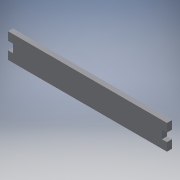
# Autodesk Inventor part: задняя
Saved by Autodesk Inventor 2019 (Build 230136000, 136)
## iProperties
Created: 2022-02-24
Part Number: задняя
Material: Типовые
Document SubType Name: Modeling
Designer: korsh
Density: 1 g/cm^3
Appearance: По умолчанию
Author: korsh
Autodesk Inventor part; units mm, degrees
ref_plane "YZ Plane" through (0, 0, 0) normal (1, 0, 0) x (0, 1, 0)
ref_plane "XZ Plane" through (0, 0, 0) normal (0, 1, 0) x (-1, 0, 0)
ref_plane "XY Plane" through (0, 0, 0) normal (0, 0, 1) x (1, 0, 0)
sketch "Эскиз1" plane through (0, 0, 0) normal (0, 0, 1) x (1, 0, 0)
  line L0 (6.072, 0) -> (186.072, 0)
  line L1 (186.072, 0) -> (186.072, -30)
  line L2 (186.072, -30) -> (6.072, -30)
  line L3 (6.072, -30) -> (6.072, 0)
  line L4 (6.072, 0) -> (0.072, 0)
  line L5 (0.072, 0) -> (0.072, -10)
  line L6 (0.072, -10) -> (6.072, -10)
  line L7 (6.072, -10) -> (6.072, 0)
  line L8 (6.072, -20) -> (0.072, -20)
  line L9 (0.072, -20) -> (0.072, -30)
  line L10 (0.072, -30) -> (6.072, -30)
  line L11 (6.072, -30) -> (6.072, -20)
  line L12 (186.072, 0) -> (192.072, 0)
  line L13 (192.072, 0) -> (192.072, -10)
  line L14 (192.072, -10) -> (186.072, -10)
  line L15 (186.072, -10) -> (186.072, 0)
  line L16 (186.072, -30) -> (186.072, -20)
  line L17 (186.072, -20) -> (192.072, -20)
  line L18 (192.072, -20) -> (192.072, -30)
  line L19 (192.072, -30) -> (186.072, -30)
  point P0 (0, 0)
  dimension "d0" = 180
  dimension "d1" = 30
  dimension "d2" = 6
  dimension "d3" = 10
  dimension "d6" = 20
  dimension "d11" = 6
  dimension "d12" = 10
  dimension "d15" = 20
  constraints: 40 end point, 6 parallel, 3 horizontal, 3 perpendicular, 2 vertical, 1 collinear, 15 other
  measures "d0" distance of L1.end L2.end
  measures "d1" distance of L0.end L1.end
  measures "d2" distance of L6.end L5.end
  measures "d3" distance of L5.end L4.end
  measures "d6" distance of L0.start L8.start
  measures "d11" distance of L13.end L14.end
  measures "d12" distance of L12.end L13.end
  measures "d15" distance of L0.end L16.end
extrude "Выдавливание1" add sketch "Эскиз1" along normal blind 6
